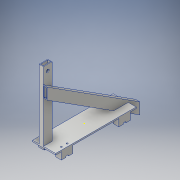
# Autodesk Inventor part: shortSupportPlate
Saved by Autodesk Inventor 2016 SP1 (Build 200210100, 210)
## iProperties
Created: 2016-02-05
Part Number: shortSupportPlate
Material: Aluminum 6061
Document SubType Name: Modeling
Designer: steele
Density: 2.7 g/cm^3
Appearance: Aluminum - Flat
Mass: 1477.33 g
Surface Area: 2861.09 cm^2
Volume: 547.159 cm^3
Author: steele
Autodesk Inventor part; units mm, degrees
ref_plane "YZ Plane" through (0, 0, 0) normal (1, 0, 0) x (0, 1, 0)
ref_plane "XZ Plane" through (0, 0, 0) normal (0, 1, 0) x (-1, 0, 0)
ref_plane "XY Plane" through (0, 0, 0) normal (0, 0, 1) x (1, 0, 0)
sketch "Sketch1" plane through (0, 0, 0) normal (0, 1, 0) x (-1, 0, 0)
  line L0 (50.8, 177.8) -> (-50.8, 177.8)
  line L1 (-50.8, 177.8) -> (-50.8, -177.8)
  line L2 (-50.8, -177.8) -> (50.8, -177.8)
  line L3 (50.8, -177.8) -> (50.8, 177.8)
  line L4 (50.8, 177.8) -> (-50.8, -177.8) construction
  line L5 (-50.8, 177.8) -> (50.8, -177.8) construction
  point P0 (0, 0)
  dimension "d0" = 355.6
  dimension "d1" = 101.6
  constraints: 12 end point, 2 midpoint, 2 parallel, 1 horizontal, 1 perpendicular
  measures "d0" distance of L2.end L0.start
  measures "d1" distance of L0.start L0.end
extrude "Extrusion1" add sketch "Sketch1" along normal blind 6.35
sketch "Sketch2" plane through (0, 6.35, 0) normal (0, 1, 0) x (1, 0, 0)
  line L0 (-50.8, -177.8) -> (50.8, -177.8) projected
  line L1 (50.8, -177.8) -> (50.8, 177.8) projected
  line L2 (50.8, 177.8) -> (-50.8, 177.8) projected
  line L3 (-50.8, 177.8) -> (-50.8, -177.8) projected
  line L4 (-50.8, -177.8) -> (50.8, -177.8) projected
  line L5 (-3.175, -177.8) -> (-22.225, -177.8)
  line L6 (-22.225, -177.8) -> (-22.225, -139.7)
  line L7 (-22.225, -139.7) -> (-3.175, -139.7)
  line L8 (-3.175, -139.7) -> (-3.175, -177.8)
  line L9 (-3.175, -177.8) -> (-22.225, -139.7) construction
  line L10 (-22.225, -177.8) -> (-3.175, -139.7) construction
  line L11 (-6.35, -174.625) -> (-6.35, -142.875)
  line L12 (-6.35, -142.875) -> (-19.05, -142.875)
  line L13 (-19.05, -142.875) -> (-19.05, -174.625)
  line L14 (-19.05, -174.625) -> (-6.35, -174.625)
  line L15 (-6.35, -174.625) -> (-19.05, -142.875) construction
  line L16 (-6.35, -142.875) -> (-19.05, -174.625) construction
  point P0 (0, 0)
  point P1 (-12.7, -158.75)
  dimension "d4" = 19.05
  dimension "d5" = 38.1
  dimension "d6" = 28.575
  dimension "d7" = 3.175
  dimension "d8" = 3.175
  constraints: 24 end point, 4 parallel, 3 midpoint, 2 perpendicular, 1 horizontal, 1 point on line, 1 vertical
  measures "d4" distance of L6.end L7.end
  measures "d5" distance of L7.end L5.start
  measures "d6" distance between parallel lines of L6 L3
  measures "d7" distance between parallel lines of L13 L6
  measures "d8" distance between parallel lines of L12 L7
extrude "Extrusion2" add sketch "Sketch2" along normal blind 304.8 contours L6 L7 L8 L0
sketch "Sketch3" plane through (-22.225, 6.35, 139.7) normal (-1, 0, 0) x (0, 0, 1)
  line L0 (38.1, 304.8) -> (0, 304.8) construction
  line L1 (19.05, 304.8) -> (19.05, 0) construction
  line L2 (-317.5, 0) -> (38.1, 0) construction
  circle A0 centre (19.05, 279.4) radius 6.35
  point P0 (-139.7, -6.35)
  dimension "d11" = 12.7
  dimension "d12" = 25.4
  constraints: 2 end point, 2 point on line, 1 centre point, 1 midpoint, 1 vertical
  measures "d11" diameter of A0
  measures "d12" distance from line of A0.centre L0
extrude "Extrusion3" cut sketch "Sketch3" against normal through all
sketch "Sketch4" plane through (0, 0, 0) normal (0, -1, 0) x (1, 0, 0)
  line L0 (-50.8, -177.8) -> (-50.8, 177.8) projected
  line L1 (-50.8, 101.6) -> (-25.4, 101.6)
  line L2 (-25.4, 101.6) -> (-25.4, 152.4)
  line L3 (-25.4, 152.4) -> (-50.8, 152.4)
  line L4 (-50.8, 152.4) -> (-50.8, 101.6)
  line L5 (-50.8, 177.8) -> (50.8, 177.8) projected
  point P0 (0, 0)
  dimension "d15" = 25.4
  dimension "d16" = 50.8
  dimension "d17" = 25.4
  constraints: 8 end point, 2 parallel, 1 horizontal, 1 perpendicular, 1 point on line
  measures "d15" distance of L2.end L3.end
  measures "d16" distance of L1.end L2.end
  measures "d17" distance between parallel lines of L5 L3
extrude "Extrusion4" add sketch "Sketch4" along normal blind 31.75
sketch "Sketch6" plane through (-50.8, 6.35, -177.8) normal (-1, 0, 0) x (0, 0, 1)
  line L0 (330.2, -38.1) -> (279.4, -38.1) projected
  circle A0 centre (304.8, -38.1) radius 6.35
  point P0 (177.8, -6.35)
  dimension "d21" = 12.7
  constraints: 1 centre point, 1 midpoint
  measures "d21" diameter of A0
extrude "Extrusion5" cut sketch "Sketch6" against normal through all
mirror "Mirror1" about plane through (0, 0, 0) normal (1, 0, 0) of "Extrusion4", "Extrusion5"
sketch "Sketch7" plane through (0, 0, 0) normal (0, -1, 0) x (1, 0, 0)
  line L0 (50.8, 177.8) -> (50.8, -177.8) projected
  line L1 (50.8, -101.6) -> (25.4, -101.6)
  line L2 (25.4, -101.6) -> (25.4, -152.4)
  line L3 (25.4, -152.4) -> (50.8, -152.4)
  line L4 (50.8, -152.4) -> (50.8, -101.6)
  line L5 (-50.8, 177.8) -> (50.8, 177.8) projected
  point P0 (0, 0)
  dimension "d24" = 279.4
  dimension "d25" = 50.8
  dimension "d26" = 25.4
  constraints: 8 end point, 2 parallel, 1 horizontal, 1 perpendicular, 1 point on line
  measures "d24" distance between parallel lines of L1 L5
  measures "d25" distance of L1.end L2.end
  measures "d26" distance of L2.end L3.end
extrude "Extrusion6" add sketch "Sketch7" along normal blind 31.75
sketch "Sketch8" plane through (50.8, 6.35, 177.8) normal (1, 0, 0) x (0, 0, -1)
  line L0 (279.4, -38.1) -> (330.2, -38.1) projected
  circle A0 centre (304.8, -38.1) radius 6.35
  point P0 (177.8, -6.35)
  dimension "d29" = 12.7
  constraints: 1 centre point, 1 midpoint
  measures "d29" diameter of A0
extrude "Extrusion7" cut sketch "Sketch8" against normal through all
mirror "Mirror2" about plane through (0, 0, 0) normal (1, 0, 0) of "Extrusion6", "Extrusion7"
sketch "Sketch9" plane through (0, 6.35, 0) normal (0, 1, 0) x (1, 0, 0)
  point P0 (38.1, -114.3)
  point P1 (38.1, -139.7)
hole "Hole1" at (38.1, 6.35, 114.3) at (38.1, 6.35, 139.7) direction (0, -1, 0) diameter 6.7564 depth 38.1
sketch "Sketch11" plane through (-3.175, 6.35, 177.8) normal (1, 0, 0) x (0, 0, -1)
  line L0 (-0.9251, 236.3733) -> (406.0956, -22.9275)
  line L1 (406.0956, -22.9275) -> (406.0956, -72.8423)
  line L2 (406.0956, -72.8423) -> (-0.9251, 186.4585)
  line L3 (-0.9251, 186.4585) -> (-0.9251, 236.3733)
  line L4 (0, 0) -> (0, 304.8) projected
  point P0 (177.8, -6.35)
  dimension "d45" = 57.5
  dimension "d48" = 482.6
  constraints: 8 end point, 3 parallel
  measures "d45" angle of L4 L2
  measures "d48" distance of L0.start L0.end
extrude "Extrusion9" add sketch "Sketch11" along normal blind 19.05
sketch "Sketch12" plane through (0, 6.35, 0) normal (0, 1, 0) x (1, 0, 0)
  point P0 (0, 0)
shell "Shell1" thickness 3.175 removed faces 1 at (3.175, 209.4468, 178.7251)
equation "\"d0\" = plateLength"
equation "\"d1\" = plateWidth"
equation "\"d2\" = plateThickness"
equation "\"d18\" = extensionSupportLength"
equation "\"d27\" = extensionSupportLength"
equation "\"plateWidth\" = 101.6"
equation "\"plateLength\" = 355.6"
equation "\"plateThickness\" = 6.35"
equation "\"extensionSupportLength\" = 31.75"
body "Solid1"
